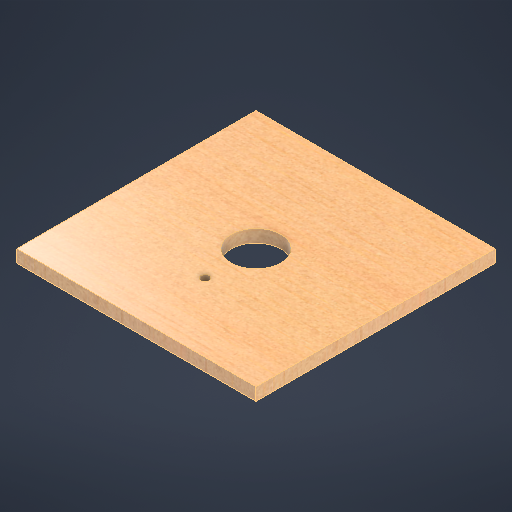
# Autodesk Inventor part: base_plate
Saved by Autodesk Inventor 2026.2 (Build 302298000, 298)
## iProperties
Created: 2026-01-14
Part Number: base_plate
Material: Pine
Document SubType Name: Modeling
Designer: User
Density: 0.570257 g/cm^3
Appearance: Yellow Pine - Solid Natural Low Gloss
Author: User
Autodesk Inventor part; units mm, degrees
ref_plane "YZ Plane" through (0, 0, 0) normal (1, 0, 0) x (0, 1, 0)
ref_plane "XZ Plane" through (0, 0, 0) normal (0, 1, 0) x (-1, 0, 0)
ref_plane "XY Plane" through (0, 0, 0) normal (0, 0, 1) x (1, 0, 0)
sketch "Sketch1" plane through (0, 0, 0) normal (0, 1, 0) x (-1, 0, 0)
  line L0 (0, 0) -> (180, 0)
  line L1 (180, 0) -> (180, -180)
  line L2 (180, -180) -> (0, -180)
  line L3 (0, -180) -> (0, 0)
  circle A0 centre (90, -90) radius 18.75
  circle A1 centre (90, -51.675) radius 3.2
  line L4 (90, -51.675) -> (90, -90) construction
  point P0 (180, -90)
  point P1 (90, -180)
  dimension "d0" = 180
  dimension "d1" = 180
  dimension "d2" = 37.5
  dimension "d3" = 0
  dimension "d4" = 0
  dimension "d5" = 6.4
  dimension "d6" = 38.325
  constraints: 10 end point, 3 parallel, 2 centre point, 2 midpoint, 1 horizontal, 1 perpendicular
  measures "d0" distance of L1.end L2.end
  measures "d1" distance of L0.end L1.end
  measures "d2" diameter of A0
  measures "d3" vertical distance of point (180, -90) L4.end
  measures "d4" horizontal distance of point (90, -180) L4.end
  measures "d5" diameter of A1
  measures "d6" distance of L4.start L4.end
extrude "Extrusion1" add sketch "Sketch1" along normal blind 9.5813
body "Solid1"
